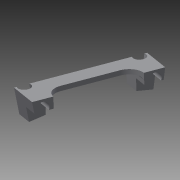
# Autodesk Inventor part: top-connector
Saved by Autodesk Inventor 2013 (Build 170138000, 138)
## iProperties
Created: 2013-09-29
Part Number: top-connector
Material: Generic
Document SubType Name: Modeling
Designer: Admin
Density: 1 g/cm^3
Author: Admin
Autodesk Inventor part; units mm, degrees
ref_plane "YZ Plane" through (0, 0, 0) normal (1, 0, 0) x (0, 1, 0)
ref_plane "XZ Plane" through (0, 0, 0) normal (0, 1, 0) x (-1, 0, 0)
ref_plane "XY Plane" through (0, 0, 0) normal (0, 0, 1) x (1, 0, 0)
ref_plane "Work Plane1" through (91.9552, 161.4495, -23.6099) normal (-0.9474155, 0.2819525, -0.1513495) x (-0.2920583, -0.9551523, 0.048847)
sketch "Sketch1" plane through (91.9552, 161.4495, -23.6099) normal (-0.9474155, 0.2819525, -0.1513495) x (-0.2920583, -0.9551523, 0.048847)
  line L0 (-20.4312, 125.2589) -> (43.1729, -264.6832) projected
  line L1 (8.25, 3.825) -> (8.25, 8.825) projected
  line L2 (8.25, 8.825) -> (-8.25, 8.825) projected
  line L3 (-8.25, 8.825) -> (-8.25, -2.6621) projected
  line L4 (-8.25, -2.6621) -> (-5.875, -2.6621) projected
  arc A0 (5.875, -2.6621) -> (-5.875, -2.6621) centre (0, 0) ccw projected
  line L5 (5.875, -2.6621) -> (8.25, -2.6621) projected
  line L6 (8.25, -2.6621) -> (8.25, 3.825) projected
  line L7 (100.25, 8.825) -> (100.25, 3.825) projected
  line L8 (100.25, 3.825) -> (100.25, -2.6621) projected
  line L9 (100.25, -2.6621) -> (102.625, -2.6621) projected
  arc A1 (114.375, -2.6621) -> (102.625, -2.6621) centre (108.5, 0) ccw projected
  line L10 (114.375, -2.6621) -> (116.75, -2.6621) projected
  line L11 (116.75, -2.6621) -> (116.75, 8.825) projected
  line L12 (116.75, 8.825) -> (100.25, 8.825) projected
  line L13 (8.25, 8.825) -> (100.25, 8.825)
  line L14 (-5.8352, -17.4665) -> (10.4496, -14.8102)
  line L15 (10.4496, -14.8102) -> (10.4496, 3.825)
  line L16 (8.25, 8.825) -> (-8.25, 8.825)
  line L17 (-8.25, 8.825) -> (-8.25, -2.6621)
  line L18 (-8.25, -2.6621) -> (-5.8352, -17.4665)
  line L19 (2.6239, -16.0867) -> (0, 0)
  line L20 (100.25, 8.825) -> (116.75, 8.825)
  line L21 (116.75, 8.825) -> (116.75, -2.6621)
  line L22 (116.75, -2.6621) -> (114.3352, -17.4665)
  line L23 (114.3352, -17.4665) -> (98.0504, -14.8102)
  line L24 (98.0504, -14.8102) -> (98.0504, 3.825)
  line L25 (98.0504, 3.825) -> (10.4496, 3.825)
  line L26 (-8.25, -2.6621) -> (-10.1237, 8.825)
  line L27 (-10.1237, 8.825) -> (-8.25, 8.825)
  line L28 (116.75, -2.6621) -> (118.6237, 8.825)
  line L29 (118.6237, 8.825) -> (116.75, 8.825)
  point P0 (182.2184, 20.728)
  dimension "d0" = 16.5
  dimension "d2" = 170.736
  dimension "d3" = 170.736
  dimension "d5" = 5
  dimension "d7" = 15
  constraints: 34 end point, 6 collinear, 6 perpendicular, 3 parallel, 2 equal length, 2 point on line
  measures "d0" distance of L14.start L14.end
  measures "d2" angle of L3 L18
  measures "d3" angle of L11 L22
  measures "d5" distance between parallel lines of L13 L25
  measures "d7" distance of L10.end L22.end
ref_plane "Work Plane3" through (60.8471, 50.6616, -35.2692) normal (-0.1761001, -0.0644633, 0.9822592) x (0.267194, 0.9572603, 0.1107254)
extrude "Extrusion1" add sketch "Sketch1" along normal blind 17.662
sketch "Sketch2" plane through (90.8404, 150.1286, -37.7212) normal (0.0820666, -0.2430656, -0.966532) x (-0.9474155, 0.2819525, -0.1513495)
  line L0 (0, 16.5) -> (0, 0) projected
  line L1 (0, 0) -> (17.662, 0) projected
  line L2 (17.662, 16.5) -> (17.662, 0) projected
  line L3 (0, 16.5) -> (17.662, 16.5) projected
  line L4 (17.6621, 16.5) -> (17.6621, 13.804)
  arc A0 (17.6621, 13.804) -> (17.6621, 2.054) centre (15, 7.929) ccw
  line L5 (17.6621, 2.054) -> (17.6621, 0)
  line L6 (17.6621, 13.804) -> (17.6621, 2.054)
  point P0 (38.0253, -175.2496)
  point P1 (15, 7.929)
  dimension "d11" = 6.45
  dimension "d13" = 11.75
  dimension "d14" = 17.6621
  constraints: 6 end point, 2 point on circle, 2 point on line, 1 centre point, 1 coincident, 1 collinear, 1 parallel, 1 perpendicular
  measures "d11" radius of A0
  measures "d13" distance of L5.start L4.end
  measures "d14" distance between parallel lines of L0 L4
extrude "Extrusion2" cut sketch "Sketch2" against normal through all contours L2 A0
sketch "Sketch3" plane through (60.8471, 50.6616, -35.2692) normal (0.1761001, 0.0644633, -0.9822592) x (-0.9474155, 0.2819525, -0.1513495)
  line L0 (17.662, 16.5) -> (17.662, 0) projected
  line L1 (0, 16.5) -> (17.662, 16.5) projected
  line L2 (0, 8.571) -> (15, 8.571)
  arc A0 (17.662, 14.446) -> (17.662, 2.6959) centre (15, 8.571) ccw
  line L3 (17.662, 14.446) -> (17.662, 2.6959)
  point P0 (38.0253, -60.8491)
  dimension "d17" = 15
  dimension "d18" = 6.45
  constraints: 4 end point, 2 point on circle, 1 centre point, 1 coincident, 1 collinear, 1 parallel, 1 point on line
  measures "d17" distance of L2.start L2.end
  measures "d18" radius of A0
extrude "Extrusion3" cut sketch "Sketch3" against normal through all
sketch "Sketch4" plane through (91.9552, 161.4495, -23.6099) normal (0.9474155, -0.2819525, 0.1513495) x (0.1307893, -0.0904813, -0.9872727)
  line L0 (-8.825, -118.6237) -> (-8.825, 10.1237) projected
  line L1 (2.6621, -116.75) -> (-8.825, -116.75) projected
  line L2 (-3.825, -98.0504) -> (14.8102, -98.0504) projected
  line L3 (14.8102, -10.4496) -> (-3.825, -10.4496) projected
  line L4 (-8.825, -8.25) -> (-3.825, -8.25) projected
  line L5 (2.6621, -8.25) -> (-3.825, -8.25) projected
  line L6 (2.6621, -5.875) -> (2.6621, -8.25) projected
  arc A0 (2.6621, 5.875) -> (2.6621, -5.875) centre (0, 0) ccw projected
  line L7 (2.6621, 8.25) -> (2.6621, 5.875) projected
  line L8 (-8.825, 8.25) -> (2.6621, 8.25) projected
  line L9 (-8.825, -8.25) -> (-8.825, 8.25) projected
  line L10 (-3.825, -100.25) -> (-8.825, -100.25) projected
  line L11 (-8.825, -116.75) -> (-8.825, -100.25) projected
  line L12 (2.6621, -116.75) -> (-8.825, -116.75) projected
  line L13 (2.6621, -114.375) -> (2.6621, -116.75) projected
  arc A1 (2.6621, -102.625) -> (2.6621, -114.375) centre (0, -108.5) ccw projected
  line L14 (2.6621, -100.25) -> (2.6621, -102.625) projected
  line L15 (-3.825, -100.25) -> (2.6621, -100.25) projected
  line L16 (2.6621, -8.25) -> (2.6621, -10.4496)
  line L17 (-3.825, -10.4496) -> (-8.825, -10.4496)
  line L18 (-3.825, -98.0504) -> (-8.825, -98.0504)
  line L19 (2.6621, -100.25) -> (2.6621, -98.0504)
  line L20 (14.8102, -98.0504) -> (17.4665, -114.3352) projected
  line L21 (-8.825, 10.1237) -> (17.4665, 5.8352) projected
  line L22 (-8.825, 8.25) -> (-8.825, 10.1237)
  line L23 (-8.825, 10.1237) -> (2.6621, 8.25)
  line L24 (2.6621, 8.25) -> (-8.825, 8.25)
  line L25 (-8.825, -116.75) -> (-8.825, -118.6237)
  line L26 (-8.825, -118.6237) -> (2.6621, -116.75)
  line L27 (2.6621, -116.75) -> (-8.825, -116.75)
  point P0 (-20.728, -182.2184)
  constraints: 20 end point, 6 perpendicular, 4 collinear, 4 point on line
extrude "Extrusion4" add sketch "Sketch4" along normal blind 15
fillet "Fillet1" radius 15 2 edges at (62.4915, 68.3687, -12.576) (88.0761, 152.0409, -16.855)
fillet "Fillet2" radius 2 4 edges at (95.5086, 149.7001, -18.1881) (80.0364, 154.3046, -20.6597) (69.9241, 66.0279, -13.909) (54.4519, 70.6324, -16.3807)
move or copy body "Move Body1" bodies to move or copy 1 copy no translate (-807.8746, 0, 0)
move or copy body "Move Body2" bodies to move or copy 1 copy no translate (0, 0, -198.7647)
ref_plane "Work Plane2" through (61.3205, 214.322, 167.5459) normal (-0.9474155, 0.2819525, -0.1513495) x (-0.2920583, -0.9551523, 0.048847)
equation "\"d3\" = d2"
body "Solid1"
